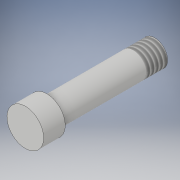
# Autodesk Inventor part: WkretDoNapinacza
Saved by Autodesk Inventor 2019 (Build 230136000, 136)
## iProperties
Created: 2020-08-27
Part Number: WkretDoNapinacza
Material: Generic
Document SubType Name: Modeling
Designer: estee
Density: 1 g/cm^3
Appearance: Default
Author: estee
Autodesk Inventor part; units mm, degrees
ref_plane "YZ Plane" through (0, 0, 0) normal (1, 0, 0) x (0, 1, 0)
ref_plane "XZ Plane" through (0, 0, 0) normal (0, 1, 0) x (-1, 0, 0)
ref_plane "XY Plane" through (0, 0, 0) normal (0, 0, 1) x (1, 0, 0)
sketch "Sketch1" plane through (0, 0, 0) normal (1, 0, 0) x (0, 1, 0)
  line L0 (0, 0) -> (4.25, 0)
  line L1 (4.25, 0) -> (4.25, -5)
  line L2 (4.25, -5) -> (3, -5)
  line L3 (3, -5) -> (3, -30)
  line L4 (3, -30) -> (0, -30)
  line L5 (0, 0) -> (0, -30)
  line L6 (0, -36) -> (0, 6) projected
  dimension "d0" = 4.25
  dimension "d1" = 1.25
  dimension "d2" = 5
  dimension "d3" = 25
  constraints: 12 end point, 4 perpendicular, 1 horizontal, 1 vertical
  measures "d0" distance of L0.start L0.end
  measures "d1" distance of L1.end L2.end
  measures "d2" distance of L0.end L1.end
  measures "d3" distance of L2.end L3.end
revolve "Revolution1" add sketch "Sketch1" angle 360 about axis through (0, 0, -10) along (0, 0, 1)
thread "Thread1" size "M6x1" class "6g" standard "ANSI Metric M Profile" length 5
body "Solid1"
